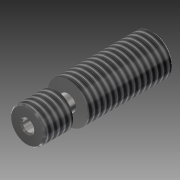
# Autodesk Inventor part: e3d_v6_heat_break
Saved by Autodesk Inventor 2013 (Build 170138000, 138)
## iProperties
Created: 2015-02-20
Part Number: e3d_v6_heat_break
Material: 一般
Document SubType Name: Modeling
Designer: Noa Izumi
Density: 1 g/cm^3
Author: Noa Izumi
Autodesk Inventor part; units mm, degrees
ref_plane "YZ Plane" through (0, 0, 0) normal (1, 0, 0) x (0, 1, 0)
ref_plane "XZ Plane" through (0, 0, 0) normal (0, 1, 0) x (-1, 0, 0)
ref_plane "XY Plane" through (0, 0, 0) normal (0, 0, 1) x (1, 0, 0)
sketch "草圖1" plane through (0, 0, 0) normal (0, 1, 0) x (-1, 0, 0)
  circle A0 centre (0, 0) radius 3
  dimension "d0" = 6
  constraints: 1 centre point, 1 coincident
  measures "d0" diameter of A0
extrude "擠出1" add sketch "草圖1" along normal blind 5
sketch "草圖2" plane through (0, 5, 0) normal (0, 1, 0) x (1, 0, 0)
  circle A0 centre (0, 0) radius 3 projected
  circle A1 centre (0, 0) radius 1.4
  dimension "d4" = 2.8
  constraints: 1 centre point, 1 coincident
  measures "d4" diameter of A1
extrude "擠出2" add sketch "草圖2" along normal blind 2.1 contours A1
sketch "草圖3" plane through (0, 7.1, 0) normal (0, 1, 0) x (1, 0, 0)
  circle A0 centre (0, 0) radius 1.4 projected
  circle A1 centre (0, 0) radius 3.5
  dimension "d8" = 7
  constraints: 1 centre point, 1 coincident
  measures "d8" diameter of A1
extrude "擠出3" add sketch "草圖3" along normal blind 14.8 contours A0 | A1
sketch "草圖5" plane through (0, 0, 0) normal (0, -1, 0) x (1, 0, 0)
  circle A0 centre (0, 0) radius 3 projected
  constraints: 1 coincident
hole "孔1" at (0, 0, 0) direction (0, 1, 0) diameter 2 end through all
chamfer "倒角2" distance 0.25 angle 45 4 edges at (3, 0, 0) (0, 0, 1) (-3.5, 21.9, 0) (0, 21.9, 1)
thread "螺紋1" size "M6x1" class "6g" standard "ANSI Metric M Profile" full length
thread "螺紋2" size "M7x1" class "6g" standard "ANSI Metric M Profile" full length
